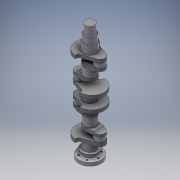
# Autodesk Inventor part: sigueñal
Saved by Autodesk Inventor 2019.3 (Build 233278000, 278)
## iProperties
Created: 2017-10-06
Part Number: sigueñal
Material: Generic
Document SubType Name: Modeling
Designer: Usuario
Density: 1 g/cm^3
Appearance: Default
Sheet Metal Rule: Default
Author: Usuario
Autodesk Inventor part; units mm, degrees
ref_plane "XZ Plane" through (0, 0, 0) normal (0, 1, 0) x (-1, 0, 0)
ref_plane "XY Plane" through (0, 0, 0) normal (0, 0, 1) x (1, 0, 0)
sketch "Sketch1" plane through (0, 0, 0) normal (0, 0, 1) x (1, 0, 0)
  circle A0 centre (0, 0) radius 21
  dimension "d0" = 42
  constraints: 1 centre point, 1 coincident
  measures "d0" diameter of A0
extrude "Extrusion1" add sketch "Sketch1" against normal blind 40
sketch "Sketch2" plane through (0, 0, -40) normal (0, 0, -1) x (-1, 0, 0)
  circle A0 centre (0, 0) radius 21 projected
  circle A1 centre (0, 0) radius 26
  dimension "d3" = 52
  constraints: 1 centre point, 1 coincident
  measures "d3" diameter of A1
extrude "Extrusion2" add sketch "Sketch2" along normal blind 29 contours A0 | A1
sketch "Sketch3" plane through (0, 0, -69) normal (0, 0, -1) x (-1, 0, 0)
  circle A0 centre (0, 0) radius 29
  dimension "d6" = 58
  constraints: 1 centre point, 1 coincident
  measures "d6" diameter of A0
extrude "Extrusion3" add sketch "Sketch3" along normal blind 34
sketch "Sketch4" plane through (0, 0, -103) normal (0, 0, -1) x (-1, 0, 0)
  circle A0 centre (0, 0) radius 32.5
  dimension "d9" = 65
  constraints: 1 centre point, 1 coincident
  measures "d9" diameter of A0
extrude "Extrusion4" add sketch "Sketch4" along normal blind 2
sketch "Sketch5" plane through (0, 0, -105) normal (0, 0, -1) x (-1, 0, 0)
  arc A0 (-51.957, 21.2586) -> (-51.957, -21.2586) centre (-45, 0) ccw
  line L0 (11.423, -42) -> (-51.957, -21.2586)
  line L1 (11.423, 42) -> (-51.957, 21.2586)
  line L2 (11.423, 0) -> (64, 0)
  arc A1 (11.423, -54.9466) -> (11.423, 54.9466) centre (9, 0) ccw
  line L3 (11.423, 54.9466) -> (11.423, 42)
  line L4 (11.423, -42) -> (11.423, -54.9466)
  point P0 (0, 0)
  dimension "d13" = 54
  dimension "d15" = 9
  dimension "d17" = 42
  constraints: 10 end point, 5 point on circle, 2 centre point, 2 vertical, 1 horizontal, 1 tangent
  measures "d13" distance of A1.centre A0.centre
  measures "d15" distance of point (0, 0) A1.centre
  measures "d17" distance of L0.start L2.start
extrude "Extrusion5" add sketch "Sketch5" along normal blind 15
sketch "Sketch6" plane through (0, 0, -120) normal (0, 0, -1) x (-1, 0, 0)
  arc A0 (-51.957, 21.2586) -> (-51.957, -21.2586) centre (-45, 0) ccw projected
  circle A1 centre (-45, 0) radius 22.368
  point P0 (0, 0)
  constraints: 1 centre point, 1 coincident, 1 concentric
extrude "Extrusion6" add sketch "Sketch6" along normal blind 2
sketch "Sketch7" plane through (45, 0, -122) normal (0, 0, -1) x (-1, 0, 0)
  circle A0 centre (0, 0) radius 22.368 projected
  circle A1 centre (0, 0) radius 21
  point P0 (45, 0)
  dimension "d22" = 42
  constraints: 1 centre point, 1 coincident
  measures "d22" diameter of A1
extrude "Extrusion7" add sketch "Sketch7" along normal blind 20 contours A1
sketch "Sketch8" plane through (45, 0, -142) normal (0, 0, -1) x (-1, 0, 0)
  circle A0 centre (0, 0) radius 21 projected
  circle A1 centre (0, 0) radius 22
  point P0 (45, 0)
  dimension "d25" = 44
  constraints: 1 centre point, 1 coincident
  measures "d25" diameter of A1
extrude "Extrusion8" add sketch "Sketch8" along normal blind 2 contours A0 | A1
sketch "Sketch9" plane through (45, 0, -144) normal (0, 0, -1) x (-1, 0, 0)
  point P0 (45, 0)
sketch "Sketch10" plane through (45, 0, -144) normal (0, 0, -1) x (-1, 0, 0)
  line L0 (-2.6889, -21.8351) -> (41.6389, -27.2938)
  line L1 (-2.6889, 21.8351) -> (41.6389, 27.2938)
  arc A0 (-2.6889, 21.8351) -> (-2.6889, -21.8351) centre (0, 0) ccw
  arc A1 (41.6389, -27.2938) -> (41.6389, 27.2938) centre (45, 0) ccw
  dimension "d29" = 27.5
  dimension "d30" = 22
  constraints: 4 end point, 4 point on circle, 2 centre point, 2 coincident, 1 tangent
  measures "d29" radius of A1
  measures "d30" radius of A0
extrude "Extrusion9" add sketch "Sketch10" along normal blind 15
sketch "Sketch11" plane through (45, 0, -159) normal (0, 0, -1) x (-1, 0, 0)
  arc A0 (41.6389, -27.2938) -> (41.6389, 27.2938) centre (45, 0) ccw projected
  circle A1 centre (45, 0) radius 27.5
  constraints: 1 centre point, 1 coincident, 1 concentric
extrude "Extrusion10" add sketch "Sketch11" along normal blind 2
ref_plane "Work Plane1" through (-27.5, 0, 0) normal (1, 0, 0) x (0, 1, 0)
ref_plane "Work Plane2" through (67, 0, 0) normal (1, 0, 0) x (0, 1, 0)
sketch "Sketch12" plane through (-27.5, 0, 0) normal (1, 0, 0) x (0, 1, 0)
  line L0 (-27.5, -161) -> (27.5, -161) projected
  line L1 (-27.2938, -144) -> (27.2938, -144) projected
  line L2 (27.2938, -144) -> (27.2938, -159) projected
  line L3 (-27.2938, -159) -> (27.2938, -159) projected
  line L4 (-27.2938, -144) -> (-27.2938, -159) projected
  line L5 (-27.5, -144) -> (27.5, -144) projected
  line L6 (-21.8351, -144) -> (21.8351, -144) projected
  line L7 (-21.8351, -144) -> (-21.8351, -159) projected
  line L8 (21.8351, -159) -> (-21.8351, -159) projected
  line L9 (21.8351, -144) -> (21.8351, -159) projected
  line L10 (22, -142) -> (-22, -142) projected
  line L11 (-35, -139) -> (35, -139)
  line L12 (35, -139) -> (35, -149)
  line L13 (35, -149) -> (-35, -149)
  line L14 (-35, -149) -> (-35, -139)
  line L15 (-35, -139) -> (35, -149) construction
  line L16 (35, -139) -> (-35, -149) construction
  point P0 (0, 0)
  point P1 (0, -144)
  dimension "d37" = 70
  dimension "d38" = 10
  constraints: 12 end point, 3 midpoint, 2 parallel, 1 horizontal, 1 perpendicular
  measures "d37" distance of L12.end L13.end
  measures "d38" distance of L11.end L12.end
extrude "Extrusion11" cut sketch "Sketch12" along normal blind 27.5 contours L4 L13 L14 L11 L12 L2 L1 | L1 L7 L13 L4 | L1 L9 L13 L7 | L1 L2 L13 L9
sketch "Sketch13" plane through (67, 0, 0) normal (1, 0, 0) x (0, 1, 0)
  line L0 (-21.8351, -159) -> (21.8351, -159) projected
  line L1 (-35, -164) -> (35, -164)
  line L2 (35, -164) -> (35, -154)
  line L3 (35, -154) -> (-35, -154)
  line L4 (-35, -154) -> (-35, -164)
  line L5 (27.2938, -159) -> (-27.2938, -159) projected
  line L6 (-35, -164) -> (35, -154) construction
  line L7 (35, -164) -> (-35, -154) construction
  point P0 (0, 0)
  point P1 (0, -159)
  dimension "d41" = 70
  dimension "d42" = 10
  constraints: 12 end point, 3 midpoint, 2 parallel, 1 horizontal, 1 perpendicular
  measures "d41" distance of L3.end L2.end
  measures "d42" distance of L2.end L1.end
extrude "Extrusion12" cut sketch "Sketch13" against normal blind 27
fillet "Fillet1" radius 10 2 edges at (0, 0, -149) (40, 0, -154)
sketch "Sketch14" plane through (0, 0, -161) normal (0, 0, -1) x (-1, 0, 0)
  circle A0 centre (0, 0) radius 27.5 projected
  circle A1 centre (0, 0) radius 26
  dimension "d46" = 52
  constraints: 1 centre point, 1 coincident
  measures "d46" diameter of A1
extrude "Extrusion13" add sketch "Sketch14" along normal blind 38.38 contours A1
sketch "Sketch15" plane through (0, 0, -199.38) normal (0, 0, -1) x (-1, 0, 0)
  circle A0 centre (0, 0) radius 26 projected
  circle A1 centre (0, 0) radius 27.5
  dimension "d49" = 55
  constraints: 1 centre point, 1 coincident
  measures "d49" diameter of A1
extrude "Extrusion14" add sketch "Sketch15" along normal blind 2 contours A0 | A1
sketch "Sketch16" plane through (0, 0, -201.38) normal (0, 0, -1) x (-1, 0, 0)
  arc A0 (47.6889, -21.8351) -> (47.6889, 21.8351) centre (45, 0) ccw
  line L0 (3.3611, 27.2938) -> (47.6889, 21.8351)
  line L1 (3.3611, -27.2938) -> (47.6889, -21.8351)
  arc A1 (3.3611, 27.2938) -> (3.3611, -27.2938) centre (0, 0) ccw
  dimension "d52" = 44
  dimension "d53" = 45
  constraints: 4 end point, 4 point on circle, 2 centre point, 1 coincident, 1 horizontal alignment, 1 tangent
  measures "d52" diameter of A0
  measures "d53" distance of A0.centre point (0, 0)
extrude "Extrusion15" add sketch "Sketch16" along normal blind 15
sketch "Sketch17" plane through (0, 0, -216.38) normal (0, 0, -1) x (-1, 0, 0)
  arc A0 (47.6889, -21.8351) -> (47.6889, 21.8351) centre (45, 0) ccw projected
  circle A1 centre (45, 0) radius 22
  point P0 (0, 0)
  dimension "d56" = 44
  constraints: 1 centre point, 1 coincident
  measures "d56" diameter of A1
extrude "Extrusion16" add sketch "Sketch17" along normal blind 2
ref_plane "Work Plane3" through (27.5, 0, 0) normal (1, 0, 0) x (0, 1, 0)
ref_plane "Work Plane4" through (-67, 0, 0) normal (1, 0, 0) x (0, 1, 0)
sketch "Sketch18" plane through (-67, 0, 0) normal (1, 0, 0) x (0, 1, 0)
  line L0 (-21.8351, -201.38) -> (21.8351, -201.38) projected
  line L1 (-35, -206.38) -> (35, -206.38)
  line L2 (35, -206.38) -> (35, -196.38)
  line L3 (35, -196.38) -> (-35, -196.38)
  line L4 (-35, -196.38) -> (-35, -206.38)
  line L5 (-35, -206.38) -> (35, -196.38) construction
  line L6 (35, -206.38) -> (-35, -196.38) construction
  point P0 (0, 0)
  point P1 (0, -201.38)
  dimension "d61" = 10
  dimension "d62" = 70
  constraints: 12 end point, 3 midpoint, 2 parallel, 1 horizontal, 1 perpendicular
  measures "d61" distance of L1.end L2.end
  measures "d62" distance of L2.end L3.end
extrude "Extrusion17" cut sketch "Sketch18" along normal blind 27.5
sketch "Sketch19" plane through (27.5, 0, 0) normal (1, 0, 0) x (0, 1, 0)
  line L0 (-27.5, -216.38) -> (27.5, -216.38) projected
  line L1 (-35, -211.38) -> (35, -211.38)
  line L2 (35, -211.38) -> (35, -221.38)
  line L3 (35, -221.38) -> (-35, -221.38)
  line L4 (-35, -221.38) -> (-35, -211.38)
  line L5 (22, -216.38) -> (-22, -216.38) projected
  line L6 (-35, -211.38) -> (35, -221.38) construction
  line L7 (35, -211.38) -> (-35, -221.38) construction
  point P0 (0, 0)
  point P1 (27.2938, -216.38)
  point P2 (-27.2938, -216.38)
  point P3 (0, -216.38)
  point P4 (-21.8351, -216.38)
  point P5 (21.8351, -216.38)
  dimension "d65" = 10
  dimension "d66" = 70
  constraints: 12 end point, 3 midpoint, 2 parallel, 1 horizontal, 1 perpendicular
  measures "d65" distance of L1.end L2.end
  measures "d66" distance of L1.start L1.end
extrude "Extrusion18" cut sketch "Sketch19" against normal blind 27
fillet "Fillet2" radius 10 2 edges at (-39.5, 0, -206.38) (0.5, 0, -211.38)
sketch "Sketch20" plane through (-45, 0, -218.38) normal (0, 0, -1) x (-1, 0, 0)
  circle A0 centre (0, 0) radius 22 projected
  circle A1 centre (0, 0) radius 21
  point P0 (-45, 0)
  dimension "d70" = 42
  constraints: 1 centre point, 1 coincident
  measures "d70" diameter of A1
extrude "Extrusion19" add sketch "Sketch20" along normal blind 20 contours A1
sketch "Sketch21" plane through (-45, 0, -238.38) normal (0, 0, -1) x (-1, 0, 0)
  circle A0 centre (0, 0) radius 21 projected
  circle A1 centre (0, 0) radius 22
  point P0 (-45, 0)
  dimension "d73" = 44
  constraints: 1 centre point, 1 coincident
  measures "d73" diameter of A1
extrude "Extrusion20" add sketch "Sketch21" along normal blind 2 contours A0 | A1
sketch "Sketch22" plane through (-45, 0, -240.38) normal (0, 0, -1) x (-1, 0, 0)
  point P0 (-45, 0)
  point P1 (0, 0)
  point P2 (-72.5, 0)
sketch "Sketch23" plane through (-45, 0, -240.38) normal (0, 0, -1) x (-1, 0, 0)
  arc A0 (7.2046, -20.7869) -> (7.2046, 20.7869) centre (0, 0) ccw
  arc A1 (-54, 55) -> (-54, -55) centre (-54, 0) ccw
  circle A2 centre (0, 0) radius 22 projected
  line L0 (7.2046, -20.7869) -> (-54, -42)
  line L1 (-120, 0) -> (34, 0)
  line L2 (7.2046, 20.7869) -> (-54, 42)
  line L3 (-54, -55) -> (-54, -42)
  line L4 (-54, 42) -> (-54, 55)
  point P0 (-45, 0)
  dimension "d82" = 110
  dimension "d85" = 54
  dimension "d88" = 42
  constraints: 10 end point, 4 point on circle, 2 centre point, 2 symmetric about line, 2 vertical, 1 coincident, 1 horizontal, 1 horizontal alignment, 1 tangent, 2 other
  measures "d82" diameter of A1
  measures "d85" distance of A0.centre A1.centre
  measures "d88" distance of L0.end A1.centre
extrude "Extrusion21" add sketch "Sketch23" along normal blind 15
fillet "Fillet3" radius 10 2 edges at (9, -42, -247.88) (9, 42, -247.88)
sketch "Sketch24" plane through (-45, 0, -255.38) normal (0, 0, -1) x (-1, 0, 0)
  arc A0 (-47.2748, -39.6691) -> (-54, -49.1177) centre (-44, -49.1177) ccw projected
  line L0 (-54, -49.1177) -> (-54, -55) projected
  arc A1 (-54, 55) -> (-54, -55) centre (-54, 0) ccw projected
  line L1 (-54, 55) -> (-54, 49.1177) projected
  arc A2 (-54, 49.1177) -> (-47.2748, 39.6691) centre (-44, 49.1177) ccw projected
  line L2 (-47.2748, 39.6691) -> (7.2046, 20.7869) projected
  arc A3 (7.2046, -20.7869) -> (7.2046, 20.7869) centre (0, 0) ccw projected
  line L3 (7.2046, -20.7869) -> (-47.2748, -39.6691) projected
  circle A4 centre (-45, 0) radius 27.5
  dimension "d92" = 55
  constraints: 1 centre point, 1 coincident
  measures "d92" diameter of A4
extrude "Extrusion22" add sketch "Sketch24" along normal blind 2 contours A4
sketch "Sketch25" plane through (0, 0, -257.38) normal (0, 0, -1) x (-1, 0, 0)
  circle A0 centre (0, 0) radius 27.5 projected
  circle A1 centre (0, 0) radius 26
  dimension "d95" = 52
  constraints: 1 centre point, 1 coincident
  measures "d95" diameter of A1
extrude "Extrusion23" add sketch "Sketch25" along normal blind 38.38 contours A1
sketch "Sketch26" plane through (0, 0, -295.76) normal (0, 0, -1) x (-1, 0, 0)
  circle A0 centre (0, 0) radius 26 projected
  circle A1 centre (0, 0) radius 27.5
  dimension "d98" = 55
  constraints: 1 centre point, 1 coincident
  measures "d98" diameter of A1
extrude "Extrusion24" add sketch "Sketch26" along normal blind 2 contours A0 | A1
sketch "Sketch27" plane through (-45, 0, -255.38) normal (0, 0, -1) x (-1, 0, 0)
  point P0 (-45, 0)
sketch "Sketch28" plane through (0, 0, -297.76) normal (0, 0, -1) x (-1, 0, 0)
  point P0 (0, 0)
ref_plane "Work Plane5" through (-45, 0, -240.38) normal (0, 0, 1) x (1, 0, 0)
ref_plane "Work Plane6" through (-45, 0, -219.19) normal (0, 0, 1) x (1, 0, 0)
ref_plane "Work Plane7" through (-45, 0, -261.57) normal (0, 0, 1) x (1, 0, 0)
ref_plane "Work Plane8" through (-45, 0, -240.38) normal (0, 0, 1) x (1, 0, 0)
sketch "Sketch29" plane through (-45, 0, -240.38) normal (0, 0, 1) x (1, 0, 0)
  point P0 (45, 0)
ref_plane "Work Plane9" through (-45, 0, -282.76) normal (0, 0, 1) x (1, 0, 0)
ref_plane "Work Plane10" through (-45, 0, -270.07) normal (0, 0, 1) x (1, 0, 0)
ref_plane "Work Plane11" through (-45, 0, -299.76) normal (0, 0, 1) x (1, 0, 0)
ref_plane "Work Plane12" through (-45, 0, -277.57) normal (0, 0, 1) x (1, 0, 0)
ref_plane "Work Plane13" through (-45, 0, -314.76) normal (0, 0, 1) x (1, 0, 0)
ref_plane "Work Plane14" through (-45, 0, -276.57) normal (0, 0, 1) x (1, 0, 0)
mirror "Mirror1" about plane through (-45, 0, -276.57) normal (0, 0, 1) of "Extrusion21", "Extrusion20", "Fillet3"
sketch "Sketch30" plane through (-45, 0, -314.76) normal (0, 0, -1) x (-1, 0, 0)
  circle A0 centre (0, 0) radius 22 projected
  circle A1 centre (0, 0) radius 21
  point P0 (-45, 0)
  dimension "d111" = 42
  constraints: 1 centre point, 1 coincident
  measures "d111" diameter of A1
extrude "Extrusion25" add sketch "Sketch30" along normal blind 20 contours A1
sketch "Sketch31" plane through (-45, 0, -334.76) normal (0, 0, -1) x (-1, 0, 0)
  circle A0 centre (0, 0) radius 21 projected
  circle A1 centre (0, 0) radius 22
  point P0 (-45, 0)
  dimension "d114" = 44
  constraints: 1 centre point, 1 coincident
  measures "d114" diameter of A1
extrude "Extrusion26" add sketch "Sketch31" along normal blind 2 contours A0 | A1
sketch "Sketch32" plane through (-45, 0, -336.76) normal (0, 0, -1) x (-1, 0, 0)
  circle A0 centre (0, 0) radius 22 projected
  arc A1 (2.6889, -21.8351) -> (2.6889, 21.8351) centre (0, 0) ccw
  line L0 (-41.6389, -27.2938) -> (2.6889, -21.8351)
  line L1 (-41.6389, 27.2938) -> (2.6889, 21.8351)
  arc A2 (-41.6389, 27.2938) -> (-41.6389, -27.2938) centre (-45, 0) ccw
  constraints: 4 end point, 4 point on circle, 4 tangent, 2 centre point, 2 coincident, 1 concentric
extrude "Extrusion27" add sketch "Sketch32" along normal blind 15
sketch "Sketch33" plane through (-45, 0, -351.76) normal (0, 0, -1) x (-1, 0, 0)
  arc A0 (-41.6389, 27.2938) -> (-41.6389, -27.2938) centre (-45, 0) ccw projected
  line L0 (-41.6389, 27.2938) -> (2.6889, 21.8351) projected
  arc A1 (2.6889, -21.8351) -> (2.6889, 21.8351) centre (0, 0) ccw projected
  line L1 (2.6889, -21.8351) -> (-41.6389, -27.2938) projected
  circle A2 centre (-45, 0) radius 27.5
  dimension "d120" = 55
  constraints: 1 centre point, 1 coincident
  measures "d120" diameter of A2
extrude "Extrusion28" add sketch "Sketch33" along normal blind 2 contours A2 A0
ref_plane "Work Plane15" through (-67, 0, 0) normal (1, 0, 0) x (0, 1, 0)
ref_plane "Work Plane16" through (27.5, 0, 0) normal (1, 0, 0) x (0, 1, 0)
sketch "Sketch34" plane through (-67, 0, 0) normal (1, 0, 0) x (0, 1, 0)
  line L0 (0, -334.76) -> (0, -351.76) projected
  line L1 (0, -297.76) -> (0, -314.76) projected
  line L2 (0, -238.38) -> (0, -255.38) projected
  line L3 (0, -206.38) -> (0, -218.38) projected
  line L4 (-35, -356.76) -> (35, -356.76)
  line L5 (35, -356.76) -> (35, -346.76)
  line L6 (35, -346.76) -> (-35, -346.76)
  line L7 (-35, -346.76) -> (-35, -356.76)
  line L8 (-35, -356.76) -> (35, -346.76) construction
  line L9 (35, -356.76) -> (-35, -346.76) construction
  point P0 (0, 0)
  dimension "d125" = 10
  dimension "d126" = 70
  constraints: 12 end point, 2 midpoint, 2 parallel, 1 horizontal, 1 perpendicular
  measures "d125" distance of L4.end L5.end
  measures "d126" distance of L4.start L4.end
extrude "Extrusion29" cut sketch "Sketch34" along normal blind 27.5
sketch "Sketch35" plane through (27.5, 0, 0) normal (1, 0, 0) x (0, 1, 0)
  line L0 (0, -336.76) -> (0, -353.76) projected
  line L1 (-51.7953, -297.76) -> (0, -297.76) projected
  line L2 (0, -297.76) -> (51.7953, -297.76) projected
  line L3 (51.7953, -297.76) -> (51.7953, -312.76) projected
  line L4 (51.7953, -312.76) -> (-51.7953, -312.76) projected
  line L5 (-51.7953, -312.76) -> (-51.7953, -297.76) projected
  line L6 (0, -295.76) -> (0, -297.76) projected
  line L7 (51.7953, -240.38) -> (51.7953, -255.38) projected
  line L8 (51.7953, -255.38) -> (0, -255.38) projected
  line L9 (0, -255.38) -> (0, -257.38) projected
  line L10 (-51.7953, -240.38) -> (51.7953, -240.38) projected
  line L11 (-51.7953, -255.38) -> (-51.7953, -240.38) projected
  line L12 (0, -255.38) -> (-51.7953, -255.38) projected
  line L13 (0, -199.38) -> (0, -211.38) projected
  line L14 (-9.206, -69) -> (9.206, -69) projected
  line L15 (9.206, -69) -> (9.206, -103) projected
  line L16 (9.206, -103) -> (17.3205, -103) projected
  line L17 (17.3205, -103) -> (17.3205, -105) projected
  line L18 (17.3205, -105) -> (29.2623, -105) projected
  line L19 (29.2623, -105) -> (29.2623, -120) projected
  line L20 (29.2623, -120) -> (13.9312, -120) projected
  line L21 (13.9312, -120) -> (13.9312, -122) projected
  line L22 (13.9312, -122) -> (11.6082, -122) projected
  line L23 (11.6082, -122) -> (11.6082, -142) projected
  line L24 (11.6082, -142) -> (13.3323, -142) projected
  line L25 (13.3323, -142) -> (13.3323, -144) projected
  line L26 (13.3323, -144) -> (24.3212, -144) projected
  line L27 (24.3212, -144) -> (24.3212, -159) projected
  line L28 (24.3212, -159) -> (0, -159) projected
  line L29 (0, -159) -> (-24.3212, -159) projected
  line L30 (-24.3212, -159) -> (-24.3212, -144) projected
  line L31 (-24.3212, -144) -> (-13.3323, -144) projected
  line L32 (-13.3323, -144) -> (-13.3323, -142) projected
  line L33 (-13.3323, -142) -> (-11.6082, -142) projected
  line L34 (-11.6082, -142) -> (-11.6082, -122) projected
  line L35 (-11.6082, -122) -> (-13.9312, -122) projected
  line L36 (-13.9312, -122) -> (-13.9312, -120) projected
  line L37 (-13.9312, -120) -> (-29.2623, -120) projected
  line L38 (-29.2623, -120) -> (-29.2623, -105) projected
  line L39 (-29.2623, -105) -> (-17.3205, -105) projected
  line L40 (-17.3205, -105) -> (-17.3205, -103) projected
  line L41 (-17.3205, -103) -> (-9.206, -103) projected
  line L42 (-9.206, -103) -> (-9.206, -69) projected
  line L43 (0, -159) -> (0, -161) projected
  line L44 (0, -336.76) -> (0, -353.76) projected
  line L45 (-51.7953, -297.76) -> (0, -297.76) projected
  line L46 (0, -297.76) -> (51.7953, -297.76) projected
  line L47 (51.7953, -297.76) -> (51.7953, -312.76) projected
  line L48 (51.7953, -312.76) -> (-51.7953, -312.76) projected
  line L49 (-51.7953, -312.76) -> (-51.7953, -297.76) projected
  line L50 (0, -295.76) -> (0, -297.76) projected
  line L51 (51.7953, -240.38) -> (51.7953, -255.38) projected
  line L52 (51.7953, -255.38) -> (0, -255.38) projected
  line L53 (0, -255.38) -> (0, -257.38) projected
  line L54 (-51.7953, -240.38) -> (51.7953, -240.38) projected
  line L55 (-51.7953, -255.38) -> (-51.7953, -240.38) projected
  line L56 (0, -255.38) -> (-51.7953, -255.38) projected
  line L57 (0, -199.38) -> (0, -211.38) projected
  line L58 (-9.206, -69) -> (9.206, -69) projected
  line L59 (9.206, -69) -> (9.206, -103) projected
  line L60 (9.206, -103) -> (17.3205, -103) projected
  line L61 (17.3205, -103) -> (17.3205, -105) projected
  line L62 (17.3205, -105) -> (29.2623, -105) projected
  line L63 (29.2623, -105) -> (29.2623, -120) projected
  line L64 (29.2623, -120) -> (13.9312, -120) projected
  line L65 (13.9312, -120) -> (13.9312, -122) projected
  line L66 (13.9312, -122) -> (11.6082, -122) projected
  line L67 (11.6082, -122) -> (11.6082, -142) projected
  line L68 (11.6082, -142) -> (13.3323, -142) projected
  line L69 (13.3323, -142) -> (13.3323, -144) projected
  line L70 (13.3323, -144) -> (24.3212, -144) projected
  line L71 (24.3212, -144) -> (24.3212, -159) projected
  line L72 (24.3212, -159) -> (0, -159) projected
  line L73 (0, -159) -> (-24.3212, -159) projected
  line L74 (-24.3212, -159) -> (-24.3212, -144) projected
  line L75 (-24.3212, -144) -> (-13.3323, -144) projected
  line L76 (-13.3323, -144) -> (-13.3323, -142) projected
  line L77 (-13.3323, -142) -> (-11.6082, -142) projected
  line L78 (-11.6082, -142) -> (-11.6082, -122) projected
  line L79 (-11.6082, -122) -> (-13.9312, -122) projected
  line L80 (-13.9312, -122) -> (-13.9312, -120) projected
  line L81 (-13.9312, -120) -> (-29.2623, -120) projected
  line L82 (-29.2623, -120) -> (-29.2623, -105) projected
  line L83 (-29.2623, -105) -> (-17.3205, -105) projected
  line L84 (-17.3205, -105) -> (-17.3205, -103) projected
  line L85 (-17.3205, -103) -> (-9.206, -103) projected
  line L86 (-9.206, -103) -> (-9.206, -69) projected
  line L87 (0, -159) -> (0, -161) projected
  line L88 (-27.5, -336.76) -> (27.5, -336.76) projected
  line L89 (35, -341.76) -> (-35, -341.76)
  line L90 (-35, -341.76) -> (-35, -331.76)
  line L91 (-35, -331.76) -> (35, -331.76)
  line L92 (35, -331.76) -> (35, -341.76)
  line L93 (35, -341.76) -> (-35, -331.76) construction
  line L94 (-35, -341.76) -> (35, -331.76) construction
  point P0 (0, 0)
  point P1 (27.2938, -336.76)
  point P2 (-27.2938, -336.76)
  dimension "d129" = 10
  dimension "d130" = 70
  constraints: 12 end point, 2 midpoint, 2 parallel, 1 horizontal, 1 perpendicular
  measures "d129" distance of L89.end L90.end
  measures "d130" distance of L89.start L89.end
extrude "Extrusion30" cut sketch "Sketch35" against normal blind 27 contours L89 L90 L91 L92
fillet "Fillet4" radius 10 2 edges at (0.5, 0, -341.76) (-39.5, 0, -346.76)
sketch "Sketch36" plane through (0, 0, -353.76) normal (0, 0, -1) x (-1, 0, 0)
  point P0 (0, 0)
sketch "Sketch37" plane through (0, 0, -353.76) normal (0, 0, -1) x (-1, 0, 0)
  circle A0 centre (0, 0) radius 27.5 projected
  circle A1 centre (0, 0) radius 26
  dimension "d134" = 52
  constraints: 1 centre point, 1 coincident
  measures "d134" diameter of A1
extrude "Extrusion31" add sketch "Sketch37" along normal blind 38.38 contours A1
sketch "Sketch38" plane through (0, 0, -392.14) normal (0, 0, -1) x (-1, 0, 0)
  circle A0 centre (0, 0) radius 26 projected
  circle A1 centre (0, 0) radius 27.5
  dimension "d137" = 55
  constraints: 1 centre point, 1 coincident
  measures "d137" diameter of A1
extrude "Extrusion32" add sketch "Sketch38" along normal blind 2 contours A0 | A1
sketch "Sketch39" plane through (0, 0, -394.14) normal (0, 0, -1) x (-1, 0, 0)
  line L0 (-3.3611, 27.2938) -> (-47.6889, 21.8351)
  line L1 (-3.3611, -27.2938) -> (-47.6889, -21.8351)
  arc A0 (-47.6889, 21.8351) -> (-47.6889, -21.8351) centre (-45, 0) ccw
  arc A1 (-3.3611, -27.2938) -> (-3.3611, 27.2938) centre (0, 0) ccw
  constraints: 4 end point, 4 point on circle, 2 centre point, 1 coincident, 1 horizontal alignment, 1 tangent
extrude "Extrusion33" add sketch "Sketch39" along normal blind 15
ref_plane "Work Plane17" through (-27.5, 0, 0) normal (1, 0, 0) x (0, 1, 0)
ref_plane "Work Plane18" through (67, 0, 0) normal (1, 0, 0) x (0, 1, 0)
sketch "Sketch40" plane through (-27.5, 0, 0) normal (1, 0, 0) x (0, 1, 0)
  line L0 (-35, -414.14) -> (35, -414.14)
  line L1 (35, -414.14) -> (35, -404.14)
  line L2 (35, -404.14) -> (-35, -404.14)
  line L3 (-35, -404.14) -> (-35, -414.14)
  line L4 (-21.8351, -409.14) -> (21.8351, -409.14) projected
  line L5 (-35, -414.14) -> (35, -404.14) construction
  line L6 (35, -414.14) -> (-35, -404.14) construction
  point P0 (0, 0)
  point P1 (0, -409.14)
  dimension "d147" = 10
  dimension "d148" = 70
  constraints: 12 end point, 3 midpoint, 2 parallel, 1 horizontal, 1 perpendicular
  measures "d147" distance of L0.end L1.end
  measures "d148" distance of L0.start L0.end
extrude "Extrusion34" cut sketch "Sketch40" along normal blind 27.5
sketch "Sketch41" plane through (67, 0, 0) normal (1, 0, 0) x (0, 1, 0)
  line L0 (0, -394.14) -> (0, -409.14) projected
  line L1 (0, -142) -> (0, -154) projected
  line L2 (-4.0407, -105) -> (4.0407, -105) projected
  line L3 (4.0407, -105) -> (4.0407, -122) projected
  line L4 (4.0407, -122) -> (-4.0407, -122) projected
  line L5 (-4.0407, -122) -> (-4.0407, -105) projected
  line L6 (35, -399.14) -> (-35, -399.14)
  line L7 (-35, -399.14) -> (-35, -389.14)
  line L8 (-35, -389.14) -> (35, -389.14)
  line L9 (35, -389.14) -> (35, -399.14)
  line L10 (35, -399.14) -> (-35, -389.14) construction
  line L11 (-35, -399.14) -> (35, -389.14) construction
  point P0 (0, 0)
  dimension "d151" = 10
  dimension "d152" = 70
  constraints: 12 end point, 2 midpoint, 2 parallel, 1 horizontal, 1 perpendicular
  measures "d151" distance of L6.end L7.end
  measures "d152" distance of L6.start L6.end
extrude "Extrusion35" cut sketch "Sketch41" against normal blind 27 contours L6 L7 L8 L9
fillet "Fillet5" radius 10 2 edges at (0, 0, -404.14) (40, 0, -399.14)
sketch "Sketch42" plane through (0, 0, -409.14) normal (0, 0, -1) x (-1, 0, 0)
  line L0 (-47.6889, 21.8351) -> (-3.3611, 27.2938) projected
  arc A0 (0, 27.5) -> (-3.3611, 27.2938) centre (0, 0) ccw projected
  line L1 (0, 27.5) -> (0, -27.5) projected
  arc A1 (-3.3611, -27.2938) -> (0, -27.5) centre (0, 0) ccw projected
  line L2 (-3.3611, -27.2938) -> (-47.6889, -21.8351) projected
  arc A2 (-47.6889, 21.8351) -> (-47.6889, -21.8351) centre (-45, 0) ccw projected
  circle A3 centre (-45, 0) radius 22
  arc A4 (-47.6889, 21.8351) -> (-47.6889, -21.8351) centre (-45, 0) ccw projected
  constraints: 1 centre point, 1 coincident, 1 concentric
extrude "Extrusion36" add sketch "Sketch42" along normal blind 2 contours A3 A2
sketch "Sketch43" plane through (45, 0, -411.14) normal (0, 0, -1) x (-1, 0, 0)
  circle A0 centre (0, 0) radius 22 projected
  circle A1 centre (0, 0) radius 21
  point P0 (45, 0)
  dimension "d158" = 42
  constraints: 1 centre point, 1 coincident
  measures "d158" diameter of A1
extrude "Extrusion37" add sketch "Sketch43" along normal blind 20 contours A1
sketch "Sketch44" plane through (45, 0, -431.14) normal (0, 0, -1) x (-1, 0, 0)
  circle A0 centre (0, 0) radius 21 projected
  circle A1 centre (0, 0) radius 22
  point P0 (45, 0)
  dimension "d161" = 44
  constraints: 1 centre point, 1 coincident
  measures "d161" diameter of A1
extrude "Extrusion38" add sketch "Sketch44" along normal blind 2 contours A0 | A1
sketch "Sketch45" plane through (45, 0, -433.14) normal (0, 0, -1) x (-1, 0, 0)
  point P0 (45, 0)
ref_plane "Work Plane22" through (0, 0, -276.57) normal (0, 0, 1) x (1, 0, 0)
ref_plane "Work Plane19" through (0, 0, -105) normal (0, 0, 1) x (1, 0, 0)
ref_plane "Work Plane21" through (45, 0, -448.14) normal (0, 0, -1) x (-1, 0, 0)
mirror "Mirror2" about plane through (0, 0, -276.57) normal (0, 0, 1) of "Extrusion5"
sketch "Sketch46" plane through (-9, 0, -448.14) normal (0, 0, -1) x (-1, 0, 0)
  line L0 (2.423, -54.9466) -> (2.423, -42) projected
  line L1 (2.423, -42) -> (-60.957, -21.2586) projected
  arc A0 (-60.957, 21.2586) -> (-60.957, -21.2586) centre (-54, 0) ccw projected
  line L2 (-60.957, 21.2586) -> (2.423, 42) projected
  line L3 (2.423, 42) -> (2.423, 54.9466) projected
  arc A1 (2.423, -54.9466) -> (2.423, 54.9466) centre (0, 0) ccw projected
  circle A2 centre (-9, 0) radius 28.5
  dimension "d167" = 57
  constraints: 1 centre point, 1 coincident
  measures "d167" diameter of A2
extrude "Extrusion39" add sketch "Sketch46" along normal blind 3 contours A2
sketch "Sketch47" plane through (0, 0, -451.14) normal (0, 0, -1) x (-1, 0, 0)
  circle A0 centre (0, 0) radius 28.5 projected
  circle A1 centre (0, 0) radius 26
  dimension "d170" = 52
  constraints: 1 centre point, 1 coincident
  measures "d170" diameter of A1
extrude "Extrusion40" add sketch "Sketch47" along normal blind 38.4 contours A1
sketch "Sketch48" plane through (0, 0, -489.54) normal (0, 0, -1) x (-1, 0, 0)
  circle A0 centre (0, 0) radius 37.5
  dimension "d173" = 75
  constraints: 1 centre point, 1 coincident
  measures "d173" diameter of A0
extrude "Extrusion41" add sketch "Sketch48" along normal blind 2
sketch "Sketch49" plane through (0, 0, -491.54) normal (0, 0, -1) x (-1, 0, 0)
  circle A0 centre (0, 0) radius 26
  dimension "d176" = 52
  constraints: 1 centre point, 1 coincident
  measures "d176" diameter of A0
extrude "Extrusion42" add sketch "Sketch49" along normal blind 20
sketch "Sketch50" plane through (0, 0, -511.54) normal (0, 0, -1) x (-1, 0, 0)
  circle A0 centre (0, 0) radius 26 projected
  circle A1 centre (0, 0) radius 50
  dimension "d179" = 100
  constraints: 1 centre point, 1 coincident
  measures "d179" diameter of A1
extrude "Extrusion43" add sketch "Sketch50" along normal blind 15 contours A0 | A1
sketch "Sketch51" plane through (0, 0, -526.54) normal (0, 0, -1) x (-1, 0, 0)
  circle A0 centre (0, 0) radius 50 projected
  line L0 (-50, 0) -> (59, 0)
  circle A1 centre (0, 0) radius 37.5 projected
  circle A2 centre (37.5, 0) radius 4
  dimension "d182" = 8
  constraints: 2 end point, 2 horizontal alignment, 1 centre point, 1 horizontal, 1 point on line, 2 other
  measures "d182" diameter of A2
extrude "Extrusion44" cut sketch "Sketch51" against normal blind 15 contours A2 A1 L0 | L0 A1 A2 | A1 A2 L0 | L0 A2 A1 picked at (38.6844, -1.0413) picked at (38.6844, 1.0413) picked at (36.19, -0.7313) picked at (36.19, 0.7313)
pattern_circular "Circular Pattern1" count 6 over 360 about axis through (0, 0, -10) along (0, 0, 1) of "Extrusion44"
fillet "Fillet6" radius 10 4 edges at (-11.423, 42, -112.5) (-11.423, 42, -440.64) (-11.423, -42, -112.5) (-11.423, -42, -440.64)
ref_plane "Work Plane20" through (45, 0, -433.14) normal (0, 0, -1) x (-1, 0, 0)
equation "\"BendRadius\" = Thickness"
equation "\"BendReliefWidth\" = Thickness"
equation "\"BendReliefDepth\" = 0.5 * Thickness"
equation "\"CornerReliefSize\" = 4 * Thickness"
equation "\"MinimumRemnant\" = 2 * Thickness"
equation "\"TransitionRadius\" = BendRadius"
equation "\"JacobiRadiusSize\" = Thickness"
equation "\"GapSize\" = Thickness"
equation "\"Thickness\" = 0.5"
body "Solid1"
